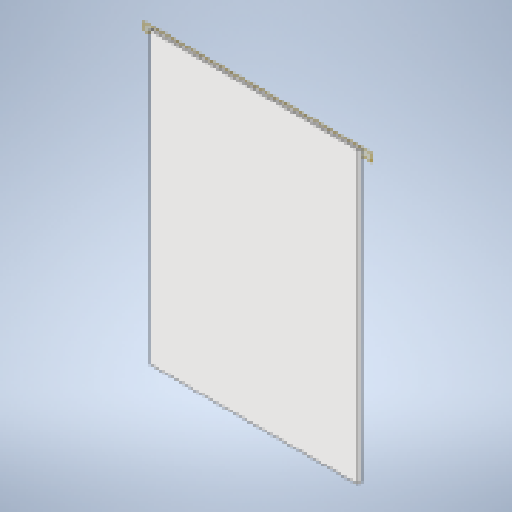
# Autodesk Inventor part: TOOLPLATE
Saved by Autodesk Inventor 2025.2 (Build 292293000, 293)
## iProperties
Created: 2026-02-10
Part Number: TOOLPLATE
Material: Generic
Document SubType Name: Modeling
Designer: composite
Density: 1 g/cm^3
Appearance: Default
Author: composite
Autodesk Inventor part; units mm, degrees
ref_plane "YZ Plane" through (0, 0, 0) normal (1, 0, 0) x (0, 1, 0)
ref_plane "XZ Plane" through (0, 0, 0) normal (0, 1, 0) x (-1, 0, 0)
ref_plane "XY Plane" through (0, 0, 0) normal (0, 0, 1) x (1, 0, 0)
ref_plane "Work Plane1" through (0, 435, 0) normal (0, 0, 1) x (1, 0, 0)
sketch "Sketch1" plane through (0, 435, 0) normal (0, 0, 1) x (1, 0, 0)
  line L0 (0, -468.8484) -> (336.5, -468.8484) projected
  line L1 (0, 0) -> (336.5, 0) projected
  line L2 (0, -471.83) -> (336.5, -471.83) projected
  line L3 (0, 3.17) -> (336.5, 3.17) projected
  line L4 (336.5, 3.17) -> (0, 3.17)
  line L5 (0, 3.17) -> (0, -471.83)
  line L6 (0, -471.83) -> (336.5, -471.83)
  line L7 (336.5, -471.83) -> (336.5, 3.17)
  line L8 (336, 2.67) -> (0.5, 2.67)
  line L9 (0.5, 2.67) -> (0.5, -471.33)
  line L10 (0.5, -471.33) -> (336, -471.33)
  line L11 (336, -471.33) -> (336, 2.67)
  point P0 (0, -435)
  point P1 (336, -468.8484)
  point P2 (336, 0)
  point P3 (0.5, 0)
  point P4 (0.5, -468.8484)
  dimension "d0" = 0.5
  constraints: 16 end point, 4 parallel, 2 perpendicular, 1 horizontal, 3 other
  measures "d0" distance between parallel lines of L7 L11
extrude "Extrusion1" add sketch "Sketch1" along normal blind 6 contours L9 L1 L11 L0 | L0 L11 L10 L9 | L9 L8 L11 L1
body "Solid1"
